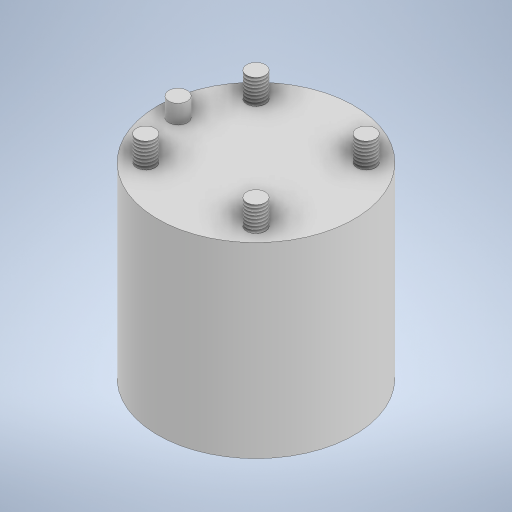
# Autodesk Inventor part: platform
Saved by Autodesk Inventor 2024.3 (Build 283343000, 343)
## iProperties
Created: 2024-11-16
Part Number: platform
Material: Generic
Document SubType Name: Modeling
Designer: Ryba
Density: 1 g/cm^3
Appearance: Default
Author: Ryba
Autodesk Inventor part; units mm, degrees
ref_plane "YZ Plane" through (0, 0, 0) normal (1, 0, 0) x (0, 1, 0)
ref_plane "XZ Plane" through (0, 0, 0) normal (0, 1, 0) x (-1, 0, 0)
ref_plane "XY Plane" through (0, 0, 0) normal (0, 0, 1) x (1, 0, 0)
sketch "Sketch4" plane through (0, 0, 0) normal (0, 1, 0) x (-1, 0, 0)
  circle A0 centre (0, 0) radius 31.5
  dimension "d7" = 63
  constraints: 1 centre point, 1 coincident
  measures "d7" diameter of A0
extrude "Extrusion4" add sketch "Sketch4" along normal blind 60
sketch "Sketch6" plane through (0, 60, 0) normal (0, 1, 0) x (1, 0, 0)
  circle A0 centre (0, 0) radius 25
  circle A1 centre (-25, 0) radius 3
  dimension "d22" = 50
  dimension "d23" = 6
  constraints: 1 centre point, 1 coincident, 1 horizontal alignment, 2 other
  measures "d23" diameter of A1
extrude "Extrusion6" add sketch "Sketch6" along normal blind 6 contours A1 A0 | A0 A1 picked at (-23.9867, 0) picked at (-25.9867, 0)
sketch "Sketch7" plane through (0, 60, 0) normal (0, 1, 0) x (1, 0, 0)
  line L0 (0, 0) -> (21.0028, 0) construction
  line L1 (0, 0) -> (25, 0) construction
  line L2 (0, 0) -> (25, 0) construction
  circle A0 centre (-17.6777, -17.6777) radius 3
  circle A1 centre (-17.6777, 17.6777) radius 3
  circle A2 centre (17.6777, 17.6777) radius 3
  circle A3 centre (17.6777, -17.6777) radius 3
  dimension "d34" = 6
  dimension "d35" = 6
  dimension "d36" = 6
  dimension "d37" = 6
  constraints: 6 end point, 4 centre point, 3 horizontal, 1 coincident
  measures "d34" diameter of A0
  measures "d35" diameter of A1
  measures "d36" diameter of A2
  measures "d37" diameter of A3
extrude "Extrusion7" add sketch "Sketch7" along normal blind 8
thread "Thread1" size "M6x1" class "6g" standard "ISO Metric profile" full length
thread "Thread2" size "M6x1" class "6g" standard "ANSI Metric M Profile" full length
thread "Thread3" size "M6x1" class "6g" standard "ANSI Metric M Profile" full length
thread "Thread4" size "M6x1" class "6g" standard "ANSI Metric M Profile" full length
sketch "Sketch8" plane through (0, 0, 0) normal (0, -1, 0) x (1, 0, 0)
  circle A0 centre (0, 0) radius 29
  constraints: 1 centre point
extrude "Extrusion8" cut sketch "Sketch8" against normal blind 36
thread "Thread5" size "M58x4" class "6H" standard "ANSI Metric M Profile" full length
sketch "Sketch9" plane through (0, 36, 0) normal (0, -1, 0) x (1, 0, 0)
  point P0 (0, 0)
thread "Thread6" size "M58x3" class "6H" standard "ANSI Metric M Profile" full length
body "Solid2"
